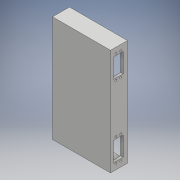
# Autodesk Inventor part: Tronco
Saved by Autodesk Inventor 2018 (Build 220112000, 112)
## iProperties
Created: 2020-03-08
Part Number: Tronco
Material: Generic
Document SubType Name: Modeling
Designer: GonzaloDiaz
Density: 1 g/cm^3
Appearance: Default
Author: GonzaloDiaz
Autodesk Inventor part; units mm, degrees
ref_plane "YZ Plane" through (0, 0, 0) normal (1, 0, 0) x (0, 1, 0)
ref_plane "XZ Plane" through (0, 0, 0) normal (0, 1, 0) x (-1, 0, 0)
ref_plane "XY Plane" through (0, 0, 0) normal (0, 0, 1) x (1, 0, 0)
sketch "servo" plane through (0, 0, 0) normal (0, 0, 1) x (1, 0, 0)
  line L0 (0, -20.0033) -> (0, 0)
  line L1 (54.4, 0) -> (54.4, -20.0033)
  line L2 (0, 0) -> (54.4, 0)
  line L3 (54.4, 0) -> (54.4, -20.0033)
  line L4 (54.4, -20.0033) -> (0, -20.0033)
  line L5 (0, -20.0033) -> (0, 0)
  circle A0 centre (3.1042, -5.0008) radius 2
  circle A1 centre (3.1042, -5.0008) radius 2
  circle A2 centre (3.1042, -15.0025) radius 2
  circle A3 centre (3.1042, -15.0025) radius 2
  circle A4 centre (51.2105, -15.0025) radius 2
  circle A5 centre (51.2105, -15.0025) radius 2
  circle A6 centre (51.2105, -5.0008) radius 2
  circle A7 centre (51.2105, -5.0008) radius 2
  line L6 (47.2, -20.0033) -> (7.2, -20.0033)
  line L7 (47.2, -20.0033) -> (7.2, -20.0033)
  line L8 (7.2, -20.0033) -> (7.2, 0)
  line L9 (7.2, 0) -> (47.2, 0)
  line L10 (47.2, 0) -> (47.2, -20.0033)
  circle A8 centre (36.7104, -10.0017) radius 2.9
  circle A9 centre (36.7104, -10.0017) radius 2.9
  point P0 (27.5156, -10.5472)
sketch "Sketch1" plane through (0, 0, 0) normal (0, 1, 0) x (-1, 0, 0)
  line L0 (0, 0) -> (120, 0)
  line L1 (120, 0) -> (120, -220)
  line L2 (120, -220) -> (0, -220)
  line L3 (0, -220) -> (0, 0)
  dimension "d0" = 120
  dimension "d1" = 220
  constraints: 8 end point, 2 parallel, 1 horizontal, 1 perpendicular
  measures "d0" distance of L1.end L2.end
  measures "d1" distance of L0.end L1.end
extrude "Extrusion1" add sketch "Sketch1" along normal blind 5
sketch "Sketch3" plane through (0, 5, 0) normal (0, 1, 0) x (1, 0, 0)
  line L0 (-120, 0) -> (0, 0) projected
  line L1 (0, 0) -> (0, 220) projected
  line L2 (-120, 0) -> (0, 0)
  line L3 (0, 0) -> (0, 220)
  line L4 (0, 220) -> (-120, 220)
  line L5 (-120, 220) -> (-120, 0)
  line L6 (-115, 5) -> (-5, 5)
  line L7 (-5, 5) -> (-5, 215)
  line L8 (-5, 215) -> (-115, 215)
  line L9 (-115, 215) -> (-115, 5)
  dimension "d4" = 5
  dimension "d5" = 5
  dimension "d6" = 5
  dimension "d7" = 5
  constraints: 16 end point, 4 parallel, 2 horizontal, 2 perpendicular
  measures "d4" distance between parallel lines of L4 L8
  measures "d5" distance between parallel lines of L0 L6
  measures "d6" distance between parallel lines of L5 L9
  measures "d7" distance between parallel lines of L1 L7
extrude "Extrusion2" add sketch "Sketch3" along normal blind 30
sketch "Sketch4" plane through (0, 0, 0) normal (1, 0, 0) x (0, 0, -1)
  line L0 (0, 0) -> (0, 35) projected
  line L1 (220, 0) -> (0, 0) projected
  line L2 (220, 0) -> (220, 35) projected
  line L3 (62.4, 26.0033) -> (62.4, 6)
  line L4 (8, 6) -> (8, 26.0033)
  line L5 (62.4, 6) -> (8, 6)
  line L6 (8, 6) -> (8, 26.0033)
  line L7 (8, 26.0033) -> (62.4, 26.0033)
  line L8 (62.4, 26.0033) -> (62.4, 6)
  circle A0 centre (59.2958, 11.0008) radius 2
  circle A1 centre (59.2958, 11.0008) radius 2
  circle A2 centre (59.2958, 21.0025) radius 2
  circle A3 centre (59.2958, 21.0025) radius 2
  circle A4 centre (11.1895, 21.0025) radius 2
  circle A5 centre (11.1895, 21.0025) radius 2
  circle A6 centre (11.1895, 11.0008) radius 2
  circle A7 centre (11.1895, 11.0008) radius 2
  line L9 (15.2, 26.0033) -> (55.2, 26.0033)
  line L10 (15.2, 26.0033) -> (55.2, 26.0033)
  line L11 (55.2, 26.0033) -> (55.2, 6)
  line L12 (55.2, 6) -> (15.2, 6)
  line L13 (15.2, 6) -> (15.2, 26.0033)
  circle A8 centre (25.6896, 16.0017) radius 2.9
  circle A9 centre (25.6896, 16.0017) radius 2.9
  line L14 (157.6, 6) -> (157.6, 26.0033)
  line L15 (212, 26.0033) -> (212, 6)
  line L16 (157.6, 26.0033) -> (212, 26.0033)
  line L17 (212, 26.0033) -> (212, 6)
  line L18 (212, 6) -> (157.6, 6)
  line L19 (157.6, 6) -> (157.6, 26.0033)
  circle A10 centre (160.7042, 21.0025) radius 2
  circle A11 centre (160.7042, 21.0025) radius 2
  circle A12 centre (160.7042, 11.0008) radius 2
  circle A13 centre (160.7042, 11.0008) radius 2
  circle A14 centre (208.8105, 11.0008) radius 2
  circle A15 centre (208.8105, 11.0008) radius 2
  circle A16 centre (208.8105, 21.0025) radius 2
  circle A17 centre (208.8105, 21.0025) radius 2
  line L20 (204.8, 6) -> (164.8, 6)
  line L21 (204.8, 6) -> (164.8, 6)
  line L22 (164.8, 6) -> (164.8, 26.0033)
  line L23 (164.8, 26.0033) -> (204.8, 26.0033)
  line L24 (204.8, 26.0033) -> (204.8, 6)
  circle A18 centre (194.3104, 16.0017) radius 2.9
  circle A19 centre (194.3104, 16.0017) radius 2.9
  dimension "d10" = 8
  dimension "d11" = 6
  dimension "d12" = 8
  dimension "d13" = 6
sketch "Sketch5" plane through (-120, 0, -220) normal (-1, 0, 0) x (0, 0, 1)
  line L0 (220, 0) -> (0, 0) projected
  line L1 (0, 0) -> (0, 35) projected
  line L2 (220, 0) -> (220, 35) projected
  line L3 (157.6, 6) -> (157.6, 26.0033)
  line L4 (212, 26.0033) -> (212, 6)
  line L5 (157.6, 26.0033) -> (212, 26.0033)
  line L6 (212, 26.0033) -> (212, 6)
  line L7 (212, 6) -> (157.6, 6)
  line L8 (157.6, 6) -> (157.6, 26.0033)
  circle A0 centre (160.7042, 21.0025) radius 2
  circle A1 centre (160.7042, 21.0025) radius 2
  circle A2 centre (160.7042, 11.0008) radius 2
  circle A3 centre (160.7042, 11.0008) radius 2
  circle A4 centre (208.8105, 11.0008) radius 2
  circle A5 centre (208.8105, 11.0008) radius 2
  circle A6 centre (208.8105, 21.0025) radius 2
  circle A7 centre (208.8105, 21.0025) radius 2
  line L9 (204.8, 6) -> (164.8, 6)
  line L10 (204.8, 6) -> (164.8, 6)
  line L11 (164.8, 6) -> (164.8, 26.0033)
  line L12 (164.8, 26.0033) -> (204.8, 26.0033)
  line L13 (204.8, 26.0033) -> (204.8, 6)
  circle A8 centre (194.3104, 16.0017) radius 2.9
  circle A9 centre (194.3104, 16.0017) radius 2.9
  line L14 (62.4, 26.0033) -> (62.4, 6)
  line L15 (8, 6) -> (8, 26.0033)
  line L16 (62.4, 6) -> (8, 6)
  line L17 (8, 6) -> (8, 26.0033)
  line L18 (8, 26.0033) -> (62.4, 26.0033)
  line L19 (62.4, 26.0033) -> (62.4, 6)
  circle A10 centre (59.2958, 11.0008) radius 2
  circle A11 centre (59.2958, 11.0008) radius 2
  circle A12 centre (59.2958, 21.0025) radius 2
  circle A13 centre (59.2958, 21.0025) radius 2
  circle A14 centre (11.1895, 21.0025) radius 2
  circle A15 centre (11.1895, 21.0025) radius 2
  circle A16 centre (11.1895, 11.0008) radius 2
  circle A17 centre (11.1895, 11.0008) radius 2
  line L20 (15.2, 26.0033) -> (55.2, 26.0033)
  line L21 (15.2, 26.0033) -> (55.2, 26.0033)
  line L22 (55.2, 26.0033) -> (55.2, 6)
  line L23 (55.2, 6) -> (15.2, 6)
  line L24 (15.2, 6) -> (15.2, 26.0033)
  circle A18 centre (25.6896, 16.0017) radius 2.9
  circle A19 centre (25.6896, 16.0017) radius 2.9
  dimension "d14" = 6
  dimension "d15" = 8
  dimension "d16" = 6
  dimension "d17" = 8
extrude "Extrusion3" cut sketch "Sketch4" against normal blind 5 contours L11 L5 L13 L7 | A0 | A2 | A4 | A6 | A8 | L22 L16 L24 L18 | A10 | A12 | A14 | A16 | A18
extrude "Extrusion4" cut sketch "Sketch5" against normal blind 5 contours L11 L5 L13 L7 | A0 | A2 | A4 | A6 | A8 | L22 L16 L24 L18 | A10 | A12 | A14 | A16 | A18
body "Solid1"
